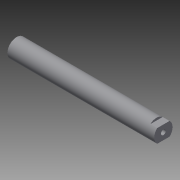
# Autodesk Inventor part: DART Rod
Saved by Autodesk Inventor 2015 (Build 190159000, 159)
## iProperties
Created: 2015-02-14
Part Number: DART Rod
Material: Generic
Document SubType Name: Modeling
Designer: pltwe4
Density: 1 g/cm^3
Appearance: Default
Author: pltwe4
Autodesk Inventor part; units mm, degrees
ref_plane "YZ Plane" through (0, 0, 0) normal (1, 0, 0) x (0, 1, 0)
ref_plane "XZ Plane" through (0, 0, 0) normal (0, 1, 0) x (-1, 0, 0)
ref_plane "XY Plane" through (0, 0, 0) normal (0, 0, 1) x (1, 0, 0)
sketch "Sketch1" plane through (0, 0, 0) normal (1, 0, 0) x (0, 1, 0)
  circle A0 centre (0, 0) radius 12.7
  dimension "d0" = 25.4
  constraints: 1 centre point, 1 coincident
  measures "d0" diameter of A0
extrude "Extrusion1" add sketch "Sketch1" along normal blind 203.2
sketch "Sketch2" plane through (203.2, 0, 0) normal (1, 0, 0) x (0, 0, -1)
  circle A0 centre (0, 0) radius 12.7 projected
  circle A1 centre (0, 0) radius 12.7 projected
  line L0 (-8.5141, 9.4234) -> (8.5141, 9.4234)
  line L1 (-8.5141, -9.4234) -> (8.5141, -9.4234)
  line L2 (-17.78, 0) -> (17.78, 0) projected
  line L3 (0, -17.78) -> (0, 17.78) projected
  circle A2 centre (0, 0) radius 3.302
  dimension "d3" = 18.8468
  dimension "d4" = 6.604
  constraints: 8 point on circle, 4 end point, 2 parallel, 1 centre point, 1 coincident, 1 other
  measures "d3" distance between parallel lines of L1 L0
  measures "d4" diameter of A2
extrude "Extrusion2" cut sketch "Sketch2" against normal blind 9.525 contours L0 L3 A0 | A0 L3 L1 | A2 L3 L2 | L2 L3 A2 | L3 L0 A0 | A0 L1 L3 | L3 A2 L2 | L2 A2 L3
body "Solid1"
